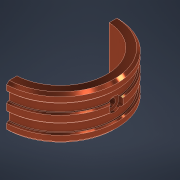
# Autodesk Inventor part: Test_Decal_Ring_Tripple
Saved by Autodesk Inventor 2022 (Build 260153000, 153)
## iProperties
Created: 2024-05-09
Part Number: Test_Decal_Ring_Tripple
Material: Generic
Document SubType Name: Modeling
Designer: jo_ki
Density: 1 g/cm^3
Appearance: Copper - Polished
Author: jo_ki
Autodesk Inventor part; units mm, degrees
ref_plane "XZ Plane" through (0, 0, 0) normal (0, 1, 0) x (-1, 0, 0)
ref_plane "XY Plane" through (0, 0, 0) normal (0, 0, 1) x (1, 0, 0)
sketch "Sketch1" plane through (0, 0, 0) normal (0, 0, 1) x (1, 0, 0)
  line L0 (18, -8.5) -> (21, -8.5)
  line L1 (21, -8.5) -> (21, 8.5)
  line L2 (21, 8.5) -> (18, 8.5)
  line L3 (18, 8.5) -> (18, -8.5)
  line L4 (18, -8.5) -> (21, 8.5) construction
  line L5 (21, -8.5) -> (18, 8.5) construction
  line L6 (21, 8.5) -> (22, 8.5)
  line L7 (22, 8.5) -> (22, 5)
  line L8 (22, 5) -> (21, 5)
  line L9 (21, 5) -> (21, 8.5)
  line L10 (21, 1.75) -> (22, 1.75)
  line L11 (22, 1.75) -> (22, -1.75)
  line L12 (22, -1.75) -> (21, -1.75)
  line L13 (21, -1.75) -> (21, 1.75)
  line L14 (21, -5) -> (22, -5)
  line L15 (22, -5) -> (22, -8.5)
  line L16 (22, -8.5) -> (21, -8.5)
  line L17 (21, -8.5) -> (21, -5)
  line L18 (-4.4, 0) -> (26.4, 0) projected
  line L19 (0, -11.9) -> (0, 11.9) projected
  point P0 (0, 0)
  point P1 (19.5, 0)
  point P2 (19.5, 0)
  dimension "d2" = 1
  dimension "d3" = 3.5
  dimension "d4" = 8.5
  dimension "d22" = 17
  dimension "d23" = 36
  dimension "d24" = 42
  constraints: 36 end point, 8 parallel, 5 point on line, 4 horizontal, 4 perpendicular, 3 collinear, 3 midpoint, 1 other
  measures "d2" distance between parallel lines of L1 L7
  measures "d3" distance between parallel lines of L12 L10
  measures "d4" distance between parallel lines of L18 L2
  measures "d22" distance between parallel lines of L0 L2
  measures "d23" diameter of L3 L19
  measures "d24" diameter of L1 L19
revolve "Revolution1" add sketch "Sketch1" angle 360 about axis through (0, -10, 0) along (0, 1, 0)
sketch "Sketch2" plane through (0, 0, 0) normal (0, 0, 1) x (1, 0, 0)
  line L0 (1, -27.8544) -> (-32.6044, -27.8544)
  line L1 (-32.6044, -27.8544) -> (-32.6044, 28.869)
  line L2 (-32.6044, 28.869) -> (1, 28.869)
  line L3 (1, 28.869) -> (1, -27.8544)
  line L4 (0, -39.1991) -> (0, 40.2136) projected
  point P0 (0, 0)
  dimension "d8" = 1
  constraints: 8 end point, 2 parallel, 1 horizontal, 1 perpendicular
  measures "d8" distance between parallel lines of L4 L3
extrude "Extrusion1" cut sketch "Sketch2" along normal through all both and the other way through all
ref_plane "Work Plane1" through (22, 0, 0) normal (1, 0, 0) x (0, 1, 0)
sketch "Sketch3" plane through (22, 0, 0) normal (1, 0, 0) x (0, 1, 0)
  point P0 (0, 0)
  point P1 (0, 0)
  constraints: 1 coincident
hole "Hole1" at (22, 0, 0) direction (-1, 0, 0) diameter 2.9 depth 5 counterbore diameter 5.5 counterbore depth 2 clearance for "Socket Head Cap Screw DIN EN ISO 4762" size "M2.5" standard "DIN"
chamfer "Chamfer1" distance 0.5 angle 45 6 edges at (15.1538, -1.75, 15.9487) (15.1538, -1.75, -15.9487) (15.1538, 1.75, 15.9487) (15.1538, 1.75, -15.9487) (22, 5, 0) (22, -5, 0)
chamfer "Chamfer2" distance 1 angle 45 2 edges at (22, 8.5, 0) (22, -8.5, 0)
body "Solid1"
